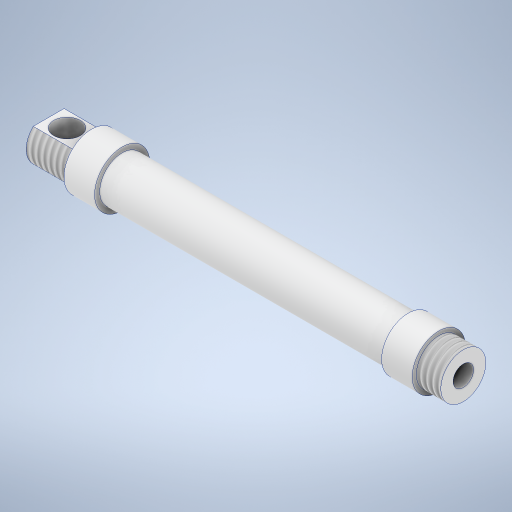
# Autodesk Inventor part: aircilinder_100_under
Saved by Autodesk Inventor 2024.1 (Build 281209000, 209)
## iProperties
Created: 2023-11-21
Part Number: aircilinder_100_under
Material: アルミニウム 6061
Document SubType Name: Modeling
Designer: haruy
Density: 2.7 g/cm^3
Appearance: アルミニウム - フラット
Author: haruy
Autodesk Inventor part; units mm, degrees
ref_plane "YZ Plane" through (0, 0, 0) normal (1, 0, 0) x (0, 1, 0)
ref_plane "XZ Plane" through (0, 0, 0) normal (0, 1, 0) x (-1, 0, 0)
ref_plane "XY Plane" through (0, 0, 0) normal (0, 0, 1) x (1, 0, 0)
sketch "スケッチ1" plane through (0, 0, 0) normal (1, 0, 0) x (0, 1, 0)
  circle A0 centre (0, 0) radius 13.5
  dimension "d0" = 27
  constraints: 1 centre point, 1 coincident
  measures "d0" diameter of A0
extrude "押し出し1" add sketch "スケッチ1" along normal blind 15
sketch "スケッチ2" plane through (15, 0, 0) normal (1, 0, 0) x (0, 0, -1)
  circle A0 centre (0, 0) radius 11
  dimension "d3" = 22
  constraints: 1 centre point, 1 coincident
  measures "d3" diameter of A0
extrude "押し出し2" add sketch "スケッチ2" along normal blind 140
sketch "スケッチ3" plane through (155, 0, 0) normal (1, 0, 0) x (0, 0, -1)
  circle A0 centre (0, 0) radius 13
  dimension "d6" = 26
  constraints: 1 centre point, 1 coincident
  measures "d6" diameter of A0
extrude "押し出し3" add sketch "スケッチ3" along normal blind 15
sketch "スケッチ4" plane through (170, 0, 0) normal (1, 0, 0) x (0, 0, -1)
  circle A0 centre (0, 0) radius 11
  dimension "d9" = 22
  constraints: 1 centre point, 1 coincident
  measures "d9" diameter of A0
extrude "押し出し4" add sketch "スケッチ4" along normal blind 12
thread "ねじ1" size "M22x3" class "6g" standard "ANSI Metric M Profile" full length
sketch "スケッチ5" plane through (0, 0, 0) normal (-1, 0, 0) x (0, 0, 1)
  circle A0 centre (0, 0) radius 11
  line L0 (7.5498, 8) -> (-7.5498, 8)
  line L1 (0, 0) -> (-11, 0)
  line L2 (7.5498, -8) -> (-7.5498, -8)
  dimension "d14" = 22
  dimension "d15" = 8
  constraints: 6 end point, 3 point on circle, 2 horizontal, 2 symmetric about line, 1 centre point, 1 coincident
  measures "d14" diameter of A0
  measures "d15" distance from line of L0 point (0, 0)
extrude "押し出し5" add sketch "スケッチ5" along normal blind 21 contours A0 L2 L0
thread "ねじ2" size "M22x3" class "6g" standard "ANSI Metric M Profile" full length
sketch "スケッチ6" plane through (0, 8, 7.5498) normal (0, 1, 0) x (1, 0, 0)
  circle A0 centre (-12, 7.5498) radius 6.5
  line L0 (-21, 0) -> (-21, 15.0997) projected
  line L1 (-21, 7.5498) -> (0, 7.5498)
  dimension "d20" = 13
  dimension "d21" = 0
  dimension "d22" = 9
  constraints: 2 end point, 1 centre point, 1 horizontal, 1 midpoint
  measures "d20" diameter of A0
  measures "d21" distance from line of L1 A0.centre
  measures "d22" distance from line of A0.centre L0
extrude "押し出し6" cut sketch "スケッチ6" against normal through all
sketch "スケッチ7" plane through (182, 0, 0) normal (1, 0, 0) x (0, 0, -1)
  circle A0 centre (0, 0) radius 5
  dimension "d25" = 10
  constraints: 1 centre point, 1 coincident
  measures "d25" diameter of A0
extrude "押し出し7" cut sketch "スケッチ7" against normal blind 100
